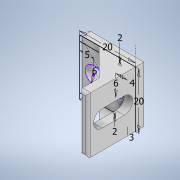
# Autodesk Inventor part: grid_board_8020_corner_mount
Saved by Autodesk Inventor 2021 (Build 250183000, 183)
## iProperties
Created: 2021-07-14
Part Number: grid_board_8020_corner_mount
Material: Generic
Document SubType Name: Modeling
Designer: Charlie
Density: 1 g/cm^3
Appearance: Default
Author: Charlie
Autodesk Inventor part; units mm, degrees
ref_plane "YZ Plane" through (0, 0, 0) normal (1, 0, 0) x (0, 1, 0)
ref_plane "XZ Plane" through (0, 0, 0) normal (0, 1, 0) x (-1, 0, 0)
ref_plane "XY Plane" through (0, 0, 0) normal (0, 0, 1) x (1, 0, 0)
sketch "Sketch1" plane through (0, 0, 0) normal (0, 0, 1) x (1, 0, 0)
  line L0 (-10, -10) -> (10, -10)
  line L1 (10, -10) -> (10, 10)
  line L2 (10, 10) -> (-10, 10)
  line L3 (-10, 10) -> (-10, -10)
  line L4 (-10, -10) -> (10, 10) construction
  line L5 (10, -10) -> (-10, 10) construction
  line L6 (7, 10) -> (7, -10)
  circle A0 centre (3, 0) radius 3
  circle A1 centre (-5, 0) radius 3
  line L7 (-5, 3) -> (3, 3)
  line L8 (-5, -3) -> (3, -3)
  line L9 (10, -10) -> (10, 17.1252) construction
  line L10 (7, 8) -> (-10, 8)
  line L11 (7, -8) -> (-10, -8)
  point P0 (0, 0)
  dimension "d0" = 20
  dimension "d1" = 20
  dimension "d2" = 3
  dimension "d3" = 6
  dimension "d4" = 4
  dimension "d5" = 6
  dimension "d6" = 5
  dimension "d16" = 2
  dimension "d17" = 2
  constraints: 24 end point, 8 point on line, 4 perpendicular, 4 point on circle, 2 centre point, 2 midpoint, 2 parallel, 1 horizontal, 1 vertical
  measures "d0" distance of L2.end L1.end
  measures "d1" distance of L1.end L0.end
  measures "d2" distance between parallel lines of L1 L6
  measures "d3" diameter of A0
  measures "d4" distance from line of L6 A0.centre
  measures "d5" diameter of A1
  measures "d6" distance from line of L3 A1.centre
  measures "d16" distance between parallel lines of L10 L2
  measures "d17" distance between parallel lines of L0 L11
extrude "Extrusion1" add sketch "Sketch1" against normal blind 3 contours L3 L11 L6 L0 | L6 L2 L1 L0 | L3 L10 L6 L11 | L3 L2 L6 L10 | A0 | A0 L8 A1 L7 | A1
extrude "Extrusion2" add sketch "Sketch1" along normal blind 17 contours L6 L2 L1 L0
sketch "Sketch2" plane through (-10, -10, -3) normal (0, -1, 0) x (1, 0, 0)
  line L0 (0, 3) -> (17, 3) projected
  line L1 (17, 3) -> (7, 3)
  line L2 (17, 3) -> (17, 20) projected
  line L3 (17, 13) -> (17, 3)
  line L4 (17, 13) -> (7, 3)
  point P0 (10, 3)
  dimension "d11" = 10
  dimension "d13" = 10
  constraints: 6 end point, 2 point on line, 1 perpendicular
  measures "d11" distance of L0.end L1.end
  measures "d13" distance of L3.start L0.end
extrude "Extrusion3" add sketch "Sketch2" against normal blind 20
extrude "Extrusion4" cut sketch "Sketch1" along normal blind 20 contours L3 L10 L6 L11 | A0 | A0 L8 A1 L7 | A1
sketch "Sketch3" plane through (7, -10, 17) normal (-1, 0, 0) x (0, 0, 1)
  circle A0 centre (-4.9998, 10.0301) radius 3
  circle A1 centre (-12.9998, 10.0301) radius 3
  line L0 (-12.9998, 13.0301) -> (-4.9998, 13.0301)
  line L1 (-12.9998, 7.0301) -> (-4.9998, 7.0301)
  line L2 (0, 20) -> (0, 0) projected
  line L3 (0, 10) -> (-2, 10) construction
  point P0 (-17, 10)
  dimension "d20" = 6
  dimension "d21" = 6
  dimension "d22" = 2
  constraints: 6 end point, 2 point on circle, 1 centre point, 1 horizontal, 1 midpoint, 5 other
  measures "d21" diameter of A1
  measures "d22" distance of L3.start L3.end
extrude "Extrusion5" cut sketch "Sketch1" against normal blind 3 contours A0 | A0 L8 A1 L7 | A1
extrude "Extrusion6" cut sketch "Sketch3" against normal blind 3
fillet "Fillet1" radius 1 8 edges at (8.5, -10, 17) (8.5, 10, 17) (7, 0, 17) (10, 0, 17) (-10, 0, 0) (-10, 0, -3) (-10, 10, -1.5) (-10, -10, -1.5)
body "Solid1"
